Autodesk Inventor part; units mm, degrees
(part 2 of 3)
ref_plane "to_Bolt_1_28_YZ" through (-253.5817, 0, -380) normal (1, 0, 0) x (0, 0, -1)
ref_plane "to_Bolt_1_28_ZX" through (-253.5817, 0, -380) normal (0, 0, -1) x (0, 1, 0)
ref_plane "to_Bolt_1_29_XY" through (-251.8625, 0, -380) normal (0, 1, 0) x (1, 0, 0)
ref_plane "to_Bolt_1_29_YZ" through (-251.8625, 0, -380) normal (1, 0, 0) x (0, 0, -1)
ref_plane "to_Bolt_1_29_ZX" through (-251.8625, 0, -380) normal (0, 0, -1) x (0, 1, 0)
ref_plane "to_Bolt_1_3_XY" through (-296.5616, 0, -380) normal (0, 1, 0) x (1, 0, 0)
ref_plane "to_Bolt_1_3_YZ" through (-296.5616, 0, -380) normal (1, 0, 0) x (0, 0, -1)
ref_plane "to_Bolt_1_3_ZX" through (-296.5616, 0, -380) normal (0, 0, -1) x (0, 1, 0)
ref_plane "to_Bolt_1_30_XY" through (-250.1433, 0, -380) normal (0, 1, 0) x (1, 0, 0)
ref_plane "to_Bolt_1_30_YZ" through (-250.1433, 0, -380) normal (1, 0, 0) x (0, 0, -1)
ref_plane "to_Bolt_1_30_ZX" through (-250.1433, 0, -380) normal (0, 0, -1) x (0, 1, 0)
ref_plane "to_Bolt_1_31_XY" through (-248.4241, 0, -380) normal (0, 1, 0) x (1, 0, 0)
ref_plane "to_Bolt_1_31_YZ" through (-248.4241, 0, -380) normal (1, 0, 0) x (0, 0, -1)
ref_plane "to_Bolt_1_31_ZX" through (-248.4241, 0, -380) normal (0, 0, -1) x (0, 1, 0)
ref_plane "to_Bolt_1_32_XY" through (-246.7049, 0, -380) normal (0, 1, 0) x (1, 0, 0)
ref_plane "to_Bolt_1_32_YZ" through (-246.7049, 0, -380) normal (1, 0, 0) x (0, 0, -1)
ref_plane "to_Bolt_1_32_ZX" through (-246.7049, 0, -380) normal (0, 0, -1) x (0, 1, 0)
ref_plane "to_Bolt_1_33_XY" through (-244.9857, 0, -380) normal (0, 1, 0) x (1, 0, 0)
ref_plane "to_Bolt_1_33_YZ" through (-244.9857, 0, -380) normal (1, 0, 0) x (0, 0, -1)
ref_plane "to_Bolt_1_33_ZX" through (-244.9857, 0, -380) normal (0, 0, -1) x (0, 1, 0)
ref_plane "to_Bolt_1_34_XY" through (-243.2665, 0, -380) normal (0, 1, 0) x (1, 0, 0)
ref_plane "to_Bolt_1_34_YZ" through (-243.2665, 0, -380) normal (1, 0, 0) x (0, 0, -1)
ref_plane "to_Bolt_1_34_ZX" through (-243.2665, 0, -380) normal (0, 0, -1) x (0, 1, 0)
ref_plane "to_Bolt_1_35_XY" through (-241.5473, 0, -380) normal (0, 1, 0) x (1, 0, 0)
ref_plane "to_Bolt_1_35_YZ" through (-241.5473, 0, -380) normal (1, 0, 0) x (0, 0, -1)
ref_plane "to_Bolt_1_35_ZX" through (-241.5473, 0, -380) normal (0, 0, -1) x (0, 1, 0)
ref_plane "to_Bolt_1_352_XY" through (-134.957, 0, 380) normal (0, 1, 0) x (1, 0, 0)
ref_plane "to_Bolt_1_352_YZ" through (-134.957, 0, 380) normal (1, 0, 0) x (0, 0, -1)
ref_plane "to_Bolt_1_352_ZX" through (-134.957, 0, 380) normal (0, 0, -1) x (0, 1, 0)
ref_plane "to_Bolt_1_353_XY" through (-133.2378, 0, 380) normal (0, 1, 0) x (1, 0, 0)
ref_plane "to_Bolt_1_353_YZ" through (-133.2378, 0, 380) normal (1, 0, 0) x (0, 0, -1)
ref_plane "to_Bolt_1_353_ZX" through (-133.2378, 0, 380) normal (0, 0, -1) x (0, 1, 0)
ref_plane "to_Bolt_1_354_XY" through (-131.5186, 0, 380) normal (0, 1, 0) x (1, 0, 0)
ref_plane "to_Bolt_1_354_YZ" through (-131.5186, 0, 380) normal (1, 0, 0) x (0, 0, -1)
ref_plane "to_Bolt_1_354_ZX" through (-131.5186, 0, 380) normal (0, 0, -1) x (0, 1, 0)
ref_plane "to_Bolt_1_355_XY" through (-129.7994, 0, 380) normal (0, 1, 0) x (1, 0, 0)
ref_plane "to_Bolt_1_355_YZ" through (-129.7994, 0, 380) normal (1, 0, 0) x (0, 0, -1)
ref_plane "to_Bolt_1_355_ZX" through (-129.7994, 0, 380) normal (0, 0, -1) x (0, 1, 0)
ref_plane "to_Bolt_1_356_XY" through (-128.0802, 0, 380) normal (0, 1, 0) x (1, 0, 0)
ref_plane "to_Bolt_1_356_YZ" through (-128.0802, 0, 380) normal (1, 0, 0) x (0, 0, -1)
ref_plane "to_Bolt_1_356_ZX" through (-128.0802, 0, 380) normal (0, 0, -1) x (0, 1, 0)
ref_plane "to_Bolt_1_357_XY" through (-126.361, 0, 380) normal (0, 1, 0) x (1, 0, 0)
ref_plane "to_Bolt_1_357_YZ" through (-126.361, 0, 380) normal (1, 0, 0) x (0, 0, -1)
ref_plane "to_Bolt_1_357_ZX" through (-126.361, 0, 380) normal (0, 0, -1) x (0, 1, 0)
ref_plane "to_Bolt_1_358_XY" through (-124.6418, 0, 380) normal (0, 1, 0) x (1, 0, 0)
ref_plane "to_Bolt_1_358_YZ" through (-124.6418, 0, 380) normal (1, 0, 0) x (0, 0, -1)
ref_plane "to_Bolt_1_358_ZX" through (-124.6418, 0, 380) normal (0, 0, -1) x (0, 1, 0)
ref_plane "to_Bolt_1_359_XY" through (-122.9226, 0, 380) normal (0, 1, 0) x (1, 0, 0)
ref_plane "to_Bolt_1_359_YZ" through (-122.9226, 0, 380) normal (1, 0, 0) x (0, 0, -1)
ref_plane "to_Bolt_1_359_ZX" through (-122.9226, 0, 380) normal (0, 0, -1) x (0, 1, 0)
ref_plane "to_Bolt_1_36_XY" through (-239.8281, 0, -380) normal (0, 1, 0) x (1, 0, 0)
ref_plane "to_Bolt_1_36_YZ" through (-239.8281, 0, -380) normal (1, 0, 0) x (0, 0, -1)
ref_plane "to_Bolt_1_36_ZX" through (-239.8281, 0, -380) normal (0, 0, -1) x (0, 1, 0)
ref_plane "to_Bolt_1_360_XY" through (-121.2034, 0, 380) normal (0, 1, 0) x (1, 0, 0)
ref_plane "to_Bolt_1_360_YZ" through (-121.2034, 0, 380) normal (1, 0, 0) x (0, 0, -1)
ref_plane "to_Bolt_1_360_ZX" through (-121.2034, 0, 380) normal (0, 0, -1) x (0, 1, 0)
ref_plane "to_Bolt_1_361_XY" through (-119.4842, 0, 380) normal (0, 1, 0) x (1, 0, 0)
ref_plane "to_Bolt_1_361_YZ" through (-119.4842, 0, 380) normal (1, 0, 0) x (0, 0, -1)
ref_plane "to_Bolt_1_361_ZX" through (-119.4842, 0, 380) normal (0, 0, -1) x (0, 1, 0)
ref_plane "to_Bolt_1_362_XY" through (-117.765, 0, 380) normal (0, 1, 0) x (1, 0, 0)
ref_plane "to_Bolt_1_362_YZ" through (-117.765, 0, 380) normal (1, 0, 0) x (0, 0, -1)
ref_plane "to_Bolt_1_362_ZX" through (-117.765, 0, 380) normal (0, 0, -1) x (0, 1, 0)
ref_plane "to_Bolt_1_363_XY" through (-116.0458, 0, 380) normal (0, 1, 0) x (1, 0, 0)
ref_plane "to_Bolt_1_363_YZ" through (-116.0458, 0, 380) normal (1, 0, 0) x (0, 0, -1)
ref_plane "to_Bolt_1_363_ZX" through (-116.0458, 0, 380) normal (0, 0, -1) x (0, 1, 0)
ref_plane "to_Bolt_1_364_XY" through (-114.3266, 0, 380) normal (0, 1, 0) x (1, 0, 0)
ref_plane "to_Bolt_1_364_YZ" through (-114.3266, 0, 380) normal (1, 0, 0) x (0, 0, -1)
ref_plane "to_Bolt_1_364_ZX" through (-114.3266, 0, 380) normal (0, 0, -1) x (0, 1, 0)
ref_plane "to_Bolt_1_365_XY" through (-112.6074, 0, 380) normal (0, 1, 0) x (1, 0, 0)
ref_plane "to_Bolt_1_365_YZ" through (-112.6074, 0, 380) normal (1, 0, 0) x (0, 0, -1)
ref_plane "to_Bolt_1_365_ZX" through (-112.6074, 0, 380) normal (0, 0, -1) x (0, 1, 0)
ref_plane "to_Bolt_1_366_XY" through (-110.8883, 0, 380) normal (0, 1, 0) x (1, 0, 0)
ref_plane "to_Bolt_1_366_YZ" through (-110.8883, 0, 380) normal (1, 0, 0) x (0, 0, -1)
ref_plane "to_Bolt_1_366_ZX" through (-110.8883, 0, 380) normal (0, 0, -1) x (0, 1, 0)
ref_plane "to_Bolt_1_367_XY" through (-109.1691, 0, 380) normal (0, 1, 0) x (1, 0, 0)
ref_plane "to_Bolt_1_367_YZ" through (-109.1691, 0, 380) normal (1, 0, 0) x (0, 0, -1)
ref_plane "to_Bolt_1_367_ZX" through (-109.1691, 0, 380) normal (0, 0, -1) x (0, 1, 0)
ref_plane "to_Bolt_1_368_XY" through (-107.4499, 0, 380) normal (0, 1, 0) x (1, 0, 0)
ref_plane "to_Bolt_1_368_YZ" through (-107.4499, 0, 380) normal (1, 0, 0) x (0, 0, -1)
ref_plane "to_Bolt_1_368_ZX" through (-107.4499, 0, 380) normal (0, 0, -1) x (0, 1, 0)
ref_plane "to_Bolt_1_369_XY" through (-105.7307, 0, 380) normal (0, 1, 0) x (1, 0, 0)
ref_plane "to_Bolt_1_369_YZ" through (-105.7307, 0, 380) normal (1, 0, 0) x (0, 0, -1)
ref_plane "to_Bolt_1_369_ZX" through (-105.7307, 0, 380) normal (0, 0, -1) x (0, 1, 0)
ref_plane "to_Bolt_1_37_XY" through (-238.1089, 0, -380) normal (0, 1, 0) x (1, 0, 0)
ref_plane "to_Bolt_1_37_YZ" through (-238.1089, 0, -380) normal (1, 0, 0) x (0, 0, -1)
ref_plane "to_Bolt_1_37_ZX" through (-238.1089, 0, -380) normal (0, 0, -1) x (0, 1, 0)
ref_plane "to_Bolt_1_370_XY" through (-104.0115, 0, 380) normal (0, 1, 0) x (1, 0, 0)
ref_plane "to_Bolt_1_370_YZ" through (-104.0115, 0, 380) normal (1, 0, 0) x (0, 0, -1)
ref_plane "to_Bolt_1_370_ZX" through (-104.0115, 0, 380) normal (0, 0, -1) x (0, 1, 0)
ref_plane "to_Bolt_1_371_XY" through (-102.2923, 0, 380) normal (0, 1, 0) x (1, 0, 0)
ref_plane "to_Bolt_1_371_YZ" through (-102.2923, 0, 380) normal (1, 0, 0) x (0, 0, -1)
ref_plane "to_Bolt_1_371_ZX" through (-102.2923, 0, 380) normal (0, 0, -1) x (0, 1, 0)
ref_plane "to_Bolt_1_372_XY" through (-100.5731, 0, 380) normal (0, 1, 0) x (1, 0, 0)
ref_plane "to_Bolt_1_372_YZ" through (-100.5731, 0, 380) normal (1, 0, 0) x (0, 0, -1)
ref_plane "to_Bolt_1_372_ZX" through (-100.5731, 0, 380) normal (0, 0, -1) x (0, 1, 0)
ref_plane "to_Bolt_1_373_XY" through (-98.8539, 0, 380) normal (0, 1, 0) x (1, 0, 0)
ref_plane "to_Bolt_1_373_YZ" through (-98.8539, 0, 380) normal (1, 0, 0) x (0, 0, -1)
ref_plane "to_Bolt_1_373_ZX" through (-98.8539, 0, 380) normal (0, 0, -1) x (0, 1, 0)
ref_plane "to_Bolt_1_374_XY" through (-97.1347, 0, 380) normal (0, 1, 0) x (1, 0, 0)
ref_plane "to_Bolt_1_374_YZ" through (-97.1347, 0, 380) normal (1, 0, 0) x (0, 0, -1)
ref_plane "to_Bolt_1_374_ZX" through (-97.1347, 0, 380) normal (0, 0, -1) x (0, 1, 0)
ref_plane "to_Bolt_1_375_XY" through (-95.4155, 0, 380) normal (0, 1, 0) x (1, 0, 0)
ref_plane "to_Bolt_1_375_YZ" through (-95.4155, 0, 380) normal (1, 0, 0) x (0, 0, -1)
ref_plane "to_Bolt_1_375_ZX" through (-95.4155, 0, 380) normal (0, 0, -1) x (0, 1, 0)
ref_plane "to_Bolt_1_376_XY" through (-93.6963, 0, 380) normal (0, 1, 0) x (1, 0, 0)
ref_plane "to_Bolt_1_376_YZ" through (-93.6963, 0, 380) normal (1, 0, 0) x (0, 0, -1)
ref_plane "to_Bolt_1_376_ZX" through (-93.6963, 0, 380) normal (0, 0, -1) x (0, 1, 0)
ref_plane "to_Bolt_1_377_XY" through (-91.9771, 0, 380) normal (0, 1, 0) x (1, 0, 0)
ref_plane "to_Bolt_1_377_YZ" through (-91.9771, 0, 380) normal (1, 0, 0) x (0, 0, -1)
ref_plane "to_Bolt_1_377_ZX" through (-91.9771, 0, 380) normal (0, 0, -1) x (0, 1, 0)
ref_plane "to_Bolt_1_378_XY" through (-90.2579, 0, 380) normal (0, 1, 0) x (1, 0, 0)
ref_plane "to_Bolt_1_378_YZ" through (-90.2579, 0, 380) normal (1, 0, 0) x (0, 0, -1)
ref_plane "to_Bolt_1_378_ZX" through (-90.2579, 0, 380) normal (0, 0, -1) x (0, 1, 0)
ref_plane "to_Bolt_1_379_XY" through (-88.5387, 0, 380) normal (0, 1, 0) x (1, 0, 0)
ref_plane "to_Bolt_1_379_YZ" through (-88.5387, 0, 380) normal (1, 0, 0) x (0, 0, -1)
ref_plane "to_Bolt_1_379_ZX" through (-88.5387, 0, 380) normal (0, 0, -1) x (0, 1, 0)
ref_plane "to_Bolt_1_38_XY" through (-236.3897, 0, -380) normal (0, 1, 0) x (1, 0, 0)
ref_plane "to_Bolt_1_38_YZ" through (-236.3897, 0, -380) normal (1, 0, 0) x (0, 0, -1)
ref_plane "to_Bolt_1_38_ZX" through (-236.3897, 0, -380) normal (0, 0, -1) x (0, 1, 0)
ref_plane "to_Bolt_1_380_XY" through (-86.8195, 0, 380) normal (0, 1, 0) x (1, 0, 0)
ref_plane "to_Bolt_1_380_YZ" through (-86.8195, 0, 380) normal (1, 0, 0) x (0, 0, -1)
ref_plane "to_Bolt_1_380_ZX" through (-86.8195, 0, 380) normal (0, 0, -1) x (0, 1, 0)
ref_plane "to_Bolt_1_381_XY" through (-85.1003, 0, 380) normal (0, 1, 0) x (1, 0, 0)
ref_plane "to_Bolt_1_381_YZ" through (-85.1003, 0, 380) normal (1, 0, 0) x (0, 0, -1)
ref_plane "to_Bolt_1_381_ZX" through (-85.1003, 0, 380) normal (0, 0, -1) x (0, 1, 0)
ref_plane "to_Bolt_1_382_XY" through (-83.3811, 0, 380) normal (0, 1, 0) x (1, 0, 0)
ref_plane "to_Bolt_1_382_YZ" through (-83.3811, 0, 380) normal (1, 0, 0) x (0, 0, -1)
ref_plane "to_Bolt_1_382_ZX" through (-83.3811, 0, 380) normal (0, 0, -1) x (0, 1, 0)
ref_plane "to_Bolt_1_383_XY" through (-81.6619, 0, 380) normal (0, 1, 0) x (1, 0, 0)
ref_plane "to_Bolt_1_383_YZ" through (-81.6619, 0, 380) normal (1, 0, 0) x (0, 0, -1)
ref_plane "to_Bolt_1_383_ZX" through (-81.6619, 0, 380) normal (0, 0, -1) x (0, 1, 0)
ref_plane "to_Bolt_1_384_XY" through (-79.9427, 0, 380) normal (0, 1, 0) x (1, 0, 0)
ref_plane "to_Bolt_1_384_YZ" through (-79.9427, 0, 380) normal (1, 0, 0) x (0, 0, -1)
ref_plane "to_Bolt_1_384_ZX" through (-79.9427, 0, 380) normal (0, 0, -1) x (0, 1, 0)
ref_plane "to_Bolt_1_385_XY" through (-78.2235, 0, 380) normal (0, 1, 0) x (1, 0, 0)
ref_plane "to_Bolt_1_385_YZ" through (-78.2235, 0, 380) normal (1, 0, 0) x (0, 0, -1)
ref_plane "to_Bolt_1_385_ZX" through (-78.2235, 0, 380) normal (0, 0, -1) x (0, 1, 0)
ref_plane "to_Bolt_1_386_XY" through (-76.5043, 0, 380) normal (0, 1, 0) x (1, 0, 0)
ref_plane "to_Bolt_1_386_YZ" through (-76.5043, 0, 380) normal (1, 0, 0) x (0, 0, -1)
ref_plane "to_Bolt_1_386_ZX" through (-76.5043, 0, 380) normal (0, 0, -1) x (0, 1, 0)
ref_plane "to_Bolt_1_387_XY" through (-74.7851, 0, 380) normal (0, 1, 0) x (1, 0, 0)
ref_plane "to_Bolt_1_387_YZ" through (-74.7851, 0, 380) normal (1, 0, 0) x (0, 0, -1)
ref_plane "to_Bolt_1_387_ZX" through (-74.7851, 0, 380) normal (0, 0, -1) x (0, 1, 0)
ref_plane "to_Bolt_1_388_XY" through (-73.0659, 0, 380) normal (0, 1, 0) x (1, 0, 0)
ref_plane "to_Bolt_1_388_YZ" through (-73.0659, 0, 380) normal (1, 0, 0) x (0, 0, -1)
ref_plane "to_Bolt_1_388_ZX" through (-73.0659, 0, 380) normal (0, 0, -1) x (0, 1, 0)
ref_plane "to_Bolt_1_389_XY" through (-71.3467, 0, 380) normal (0, 1, 0) x (1, 0, 0)
ref_plane "to_Bolt_1_389_YZ" through (-71.3467, 0, 380) normal (1, 0, 0) x (0, 0, -1)
ref_plane "to_Bolt_1_389_ZX" through (-71.3467, 0, 380) normal (0, 0, -1) x (0, 1, 0)
ref_plane "to_Bolt_1_39_XY" through (-234.6705, 0, -380) normal (0, 1, 0) x (1, 0, 0)
ref_plane "to_Bolt_1_39_YZ" through (-234.6705, 0, -380) normal (1, 0, 0) x (0, 0, -1)
ref_plane "to_Bolt_1_39_ZX" through (-234.6705, 0, -380) normal (0, 0, -1) x (0, 1, 0)
ref_plane "to_Bolt_1_390_XY" through (-69.6275, 0, 380) normal (0, 1, 0) x (1, 0, 0)
ref_plane "to_Bolt_1_390_YZ" through (-69.6275, 0, 380) normal (1, 0, 0) x (0, 0, -1)
ref_plane "to_Bolt_1_390_ZX" through (-69.6275, 0, 380) normal (0, 0, -1) x (0, 1, 0)
ref_plane "to_Bolt_1_391_XY" through (-67.9083, 0, 380) normal (0, 1, 0) x (1, 0, 0)
ref_plane "to_Bolt_1_391_YZ" through (-67.9083, 0, 380) normal (1, 0, 0) x (0, 0, -1)
ref_plane "to_Bolt_1_391_ZX" through (-67.9083, 0, 380) normal (0, 0, -1) x (0, 1, 0)
ref_plane "to_Bolt_1_392_XY" through (-66.1891, 0, 380) normal (0, 1, 0) x (1, 0, 0)
ref_plane "to_Bolt_1_392_YZ" through (-66.1891, 0, 380) normal (1, 0, 0) x (0, 0, -1)
ref_plane "to_Bolt_1_392_ZX" through (-66.1891, 0, 380) normal (0, 0, -1) x (0, 1, 0)
ref_plane "to_Bolt_1_393_XY" through (-64.4699, 0, 380) normal (0, 1, 0) x (1, 0, 0)
ref_plane "to_Bolt_1_393_YZ" through (-64.4699, 0, 380) normal (1, 0, 0) x (0, 0, -1)
ref_plane "to_Bolt_1_393_ZX" through (-64.4699, 0, 380) normal (0, 0, -1) x (0, 1, 0)
ref_plane "to_Bolt_1_394_XY" through (-62.7507, 0, 380) normal (0, 1, 0) x (1, 0, 0)
ref_plane "to_Bolt_1_394_YZ" through (-62.7507, 0, 380) normal (1, 0, 0) x (0, 0, -1)
ref_plane "to_Bolt_1_394_ZX" through (-62.7507, 0, 380) normal (0, 0, -1) x (0, 1, 0)
ref_plane "to_Bolt_1_395_XY" through (-61.0315, 0, 380) normal (0, 1, 0) x (1, 0, 0)
ref_plane "to_Bolt_1_395_YZ" through (-61.0315, 0, 380) normal (1, 0, 0) x (0, 0, -1)
ref_plane "to_Bolt_1_395_ZX" through (-61.0315, 0, 380) normal (0, 0, -1) x (0, 1, 0)
ref_plane "to_Bolt_1_396_XY" through (-59.3123, 0, 380) normal (0, 1, 0) x (1, 0, 0)
ref_plane "to_Bolt_1_396_YZ" through (-59.3123, 0, 380) normal (1, 0, 0) x (0, 0, -1)
ref_plane "to_Bolt_1_396_ZX" through (-59.3123, 0, 380) normal (0, 0, -1) x (0, 1, 0)
ref_plane "to_Bolt_1_397_XY" through (-57.5931, 0, 380) normal (0, 1, 0) x (1, 0, 0)
ref_plane "to_Bolt_1_397_YZ" through (-57.5931, 0, 380) normal (1, 0, 0) x (0, 0, -1)
ref_plane "to_Bolt_1_397_ZX" through (-57.5931, 0, 380) normal (0, 0, -1) x (0, 1, 0)
ref_plane "to_Bolt_1_398_XY" through (-55.8739, 0, 380) normal (0, 1, 0) x (1, 0, 0)
ref_plane "to_Bolt_1_398_YZ" through (-55.8739, 0, 380) normal (1, 0, 0) x (0, 0, -1)
ref_plane "to_Bolt_1_398_ZX" through (-55.8739, 0, 380) normal (0, 0, -1) x (0, 1, 0)
ref_plane "to_Bolt_1_399_XY" through (-54.1547, 0, 380) normal (0, 1, 0) x (1, 0, 0)
ref_plane "to_Bolt_1_399_YZ" through (-54.1547, 0, 380) normal (1, 0, 0) x (0, 0, -1)
ref_plane "to_Bolt_1_399_ZX" through (-54.1547, 0, 380) normal (0, 0, -1) x (0, 1, 0)
ref_plane "to_Bolt_1_4_XY" through (-294.8424, 0, -380) normal (0, 1, 0) x (1, 0, 0)
ref_plane "to_Bolt_1_4_YZ" through (-294.8424, 0, -380) normal (1, 0, 0) x (0, 0, -1)
ref_plane "to_Bolt_1_4_ZX" through (-294.8424, 0, -380) normal (0, 0, -1) x (0, 1, 0)
ref_plane "to_Bolt_1_40_XY" through (-232.9513, 0, -380) normal (0, 1, 0) x (1, 0, 0)
ref_plane "to_Bolt_1_40_YZ" through (-232.9513, 0, -380) normal (1, 0, 0) x (0, 0, -1)
ref_plane "to_Bolt_1_40_ZX" through (-232.9513, 0, -380) normal (0, 0, -1) x (0, 1, 0)
ref_plane "to_Bolt_1_400_XY" through (-52.4355, 0, 380) normal (0, 1, 0) x (1, 0, 0)
ref_plane "to_Bolt_1_400_YZ" through (-52.4355, 0, 380) normal (1, 0, 0) x (0, 0, -1)
ref_plane "to_Bolt_1_400_ZX" through (-52.4355, 0, 380) normal (0, 0, -1) x (0, 1, 0)
ref_plane "to_Bolt_1_401_XY" through (-50.7163, 0, 380) normal (0, 1, 0) x (1, 0, 0)
ref_plane "to_Bolt_1_401_YZ" through (-50.7163, 0, 380) normal (1, 0, 0) x (0, 0, -1)
ref_plane "to_Bolt_1_401_ZX" through (-50.7163, 0, 380) normal (0, 0, -1) x (0, 1, 0)
ref_plane "to_Bolt_1_402_XY" through (-48.9971, 0, 380) normal (0, 1, 0) x (1, 0, 0)
ref_plane "to_Bolt_1_402_YZ" through (-48.9971, 0, 380) normal (1, 0, 0) x (0, 0, -1)
ref_plane "to_Bolt_1_402_ZX" through (-48.9971, 0, 380) normal (0, 0, -1) x (0, 1, 0)
ref_plane "to_Bolt_1_403_XY" through (-47.2779, 0, 380) normal (0, 1, 0) x (1, 0, 0)
ref_plane "to_Bolt_1_403_YZ" through (-47.2779, 0, 380) normal (1, 0, 0) x (0, 0, -1)
ref_plane "to_Bolt_1_403_ZX" through (-47.2779, 0, 380) normal (0, 0, -1) x (0, 1, 0)
ref_plane "to_Bolt_1_404_XY" through (-45.5587, 0, 380) normal (0, 1, 0) x (1, 0, 0)
ref_plane "to_Bolt_1_404_YZ" through (-45.5587, 0, 380) normal (1, 0, 0) x (0, 0, -1)
ref_plane "to_Bolt_1_404_ZX" through (-45.5587, 0, 380) normal (0, 0, -1) x (0, 1, 0)
ref_plane "to_Bolt_1_405_XY" through (-43.8395, 0, 380) normal (0, 1, 0) x (1, 0, 0)
ref_plane "to_Bolt_1_405_YZ" through (-43.8395, 0, 380) normal (1, 0, 0) x (0, 0, -1)
ref_plane "to_Bolt_1_405_ZX" through (-43.8395, 0, 380) normal (0, 0, -1) x (0, 1, 0)
ref_plane "to_Bolt_1_406_XY" through (-42.1203, 0, 380) normal (0, 1, 0) x (1, 0, 0)
ref_plane "to_Bolt_1_406_YZ" through (-42.1203, 0, 380) normal (1, 0, 0) x (0, 0, -1)
ref_plane "to_Bolt_1_406_ZX" through (-42.1203, 0, 380) normal (0, 0, -1) x (0, 1, 0)
ref_plane "to_Bolt_1_407_XY" through (-40.4011, 0, 380) normal (0, 1, 0) x (1, 0, 0)
ref_plane "to_Bolt_1_407_YZ" through (-40.4011, 0, 380) normal (1, 0, 0) x (0, 0, -1)
ref_plane "to_Bolt_1_407_ZX" through (-40.4011, 0, 380) normal (0, 0, -1) x (0, 1, 0)
ref_plane "to_Bolt_1_408_XY" through (-38.6819, 0, 380) normal (0, 1, 0) x (1, 0, 0)
ref_plane "to_Bolt_1_408_YZ" through (-38.6819, 0, 380) normal (1, 0, 0) x (0, 0, -1)
ref_plane "to_Bolt_1_408_ZX" through (-38.6819, 0, 380) normal (0, 0, -1) x (0, 1, 0)
ref_plane "to_Bolt_1_409_XY" through (-36.9628, 0, 380) normal (0, 1, 0) x (1, 0, 0)
ref_plane "to_Bolt_1_409_YZ" through (-36.9628, 0, 380) normal (1, 0, 0) x (0, 0, -1)
ref_plane "to_Bolt_1_409_ZX" through (-36.9628, 0, 380) normal (0, 0, -1) x (0, 1, 0)
ref_plane "to_Bolt_1_41_XY" through (-231.2321, 0, -380) normal (0, 1, 0) x (1, 0, 0)
ref_plane "to_Bolt_1_41_YZ" through (-231.2321, 0, -380) normal (1, 0, 0) x (0, 0, -1)
ref_plane "to_Bolt_1_41_ZX" through (-231.2321, 0, -380) normal (0, 0, -1) x (0, 1, 0)
ref_plane "to_Bolt_1_410_XY" through (-35.2436, 0, 380) normal (0, 1, 0) x (1, 0, 0)
ref_plane "to_Bolt_1_410_YZ" through (-35.2436, 0, 380) normal (1, 0, 0) x (0, 0, -1)
ref_plane "to_Bolt_1_410_ZX" through (-35.2436, 0, 380) normal (0, 0, -1) x (0, 1, 0)
ref_plane "to_Bolt_1_411_XY" through (-33.5244, 0, 380) normal (0, 1, 0) x (1, 0, 0)
ref_plane "to_Bolt_1_411_YZ" through (-33.5244, 0, 380) normal (1, 0, 0) x (0, 0, -1)
ref_plane "to_Bolt_1_411_ZX" through (-33.5244, 0, 380) normal (0, 0, -1) x (0, 1, 0)
ref_plane "to_Bolt_1_412_XY" through (-31.8052, 0, 380) normal (0, 1, 0) x (1, 0, 0)
ref_plane "to_Bolt_1_412_YZ" through (-31.8052, 0, 380) normal (1, 0, 0) x (0, 0, -1)
ref_plane "to_Bolt_1_412_ZX" through (-31.8052, 0, 380) normal (0, 0, -1) x (0, 1, 0)
ref_plane "to_Bolt_1_413_XY" through (-30.086, 0, 380) normal (0, 1, 0) x (1, 0, 0)
ref_plane "to_Bolt_1_413_YZ" through (-30.086, 0, 380) normal (1, 0, 0) x (0, 0, -1)
ref_plane "to_Bolt_1_413_ZX" through (-30.086, 0, 380) normal (0, 0, -1) x (0, 1, 0)
ref_plane "to_Bolt_1_414_XY" through (-28.3668, 0, 380) normal (0, 1, 0) x (1, 0, 0)
ref_plane "to_Bolt_1_414_YZ" through (-28.3668, 0, 380) normal (1, 0, 0) x (0, 0, -1)
ref_plane "to_Bolt_1_414_ZX" through (-28.3668, 0, 380) normal (0, 0, -1) x (0, 1, 0)
ref_plane "to_Bolt_1_415_XY" through (-26.6476, 0, 380) normal (0, 1, 0) x (1, 0, 0)
ref_plane "to_Bolt_1_415_YZ" through (-26.6476, 0, 380) normal (1, 0, 0) x (0, 0, -1)
ref_plane "to_Bolt_1_415_ZX" through (-26.6476, 0, 380) normal (0, 0, -1) x (0, 1, 0)
ref_plane "to_Bolt_1_416_XY" through (-24.9284, 0, 380) normal (0, 1, 0) x (1, 0, 0)
ref_plane "to_Bolt_1_416_YZ" through (-24.9284, 0, 380) normal (1, 0, 0) x (0, 0, -1)
ref_plane "to_Bolt_1_416_ZX" through (-24.9284, 0, 380) normal (0, 0, -1) x (0, 1, 0)
ref_plane "to_Bolt_1_417_XY" through (-23.2092, 0, 380) normal (0, 1, 0) x (1, 0, 0)
ref_plane "to_Bolt_1_417_YZ" through (-23.2092, 0, 380) normal (1, 0, 0) x (0, 0, -1)
ref_plane "to_Bolt_1_417_ZX" through (-23.2092, 0, 380) normal (0, 0, -1) x (0, 1, 0)
ref_plane "to_Bolt_1_418_XY" through (-21.49, 0, 380) normal (0, 1, 0) x (1, 0, 0)
ref_plane "to_Bolt_1_418_YZ" through (-21.49, 0, 380) normal (1, 0, 0) x (0, 0, -1)
ref_plane "to_Bolt_1_418_ZX" through (-21.49, 0, 380) normal (0, 0, -1) x (0, 1, 0)
ref_plane "to_Bolt_1_419_XY" through (-19.7708, 0, 380) normal (0, 1, 0) x (1, 0, 0)
ref_plane "to_Bolt_1_419_YZ" through (-19.7708, 0, 380) normal (1, 0, 0) x (0, 0, -1)
ref_plane "to_Bolt_1_419_ZX" through (-19.7708, 0, 380) normal (0, 0, -1) x (0, 1, 0)
ref_plane "to_Bolt_1_42_XY" through (-229.5129, 0, -380) normal (0, 1, 0) x (1, 0, 0)
ref_plane "to_Bolt_1_42_YZ" through (-229.5129, 0, -380) normal (1, 0, 0) x (0, 0, -1)
ref_plane "to_Bolt_1_42_ZX" through (-229.5129, 0, -380) normal (0, 0, -1) x (0, 1, 0)
ref_plane "to_Bolt_1_420_XY" through (-18.0516, 0, 380) normal (0, 1, 0) x (1, 0, 0)
ref_plane "to_Bolt_1_420_YZ" through (-18.0516, 0, 380) normal (1, 0, 0) x (0, 0, -1)
ref_plane "to_Bolt_1_420_ZX" through (-18.0516, 0, 380) normal (0, 0, -1) x (0, 1, 0)
ref_plane "to_Bolt_1_421_XY" through (-16.3324, 0, 380) normal (0, 1, 0) x (1, 0, 0)
ref_plane "to_Bolt_1_421_YZ" through (-16.3324, 0, 380) normal (1, 0, 0) x (0, 0, -1)
ref_plane "to_Bolt_1_421_ZX" through (-16.3324, 0, 380) normal (0, 0, -1) x (0, 1, 0)
ref_plane "to_Bolt_1_422_XY" through (-14.6132, 0, 380) normal (0, 1, 0) x (1, 0, 0)
ref_plane "to_Bolt_1_422_YZ" through (-14.6132, 0, 380) normal (1, 0, 0) x (0, 0, -1)
ref_plane "to_Bolt_1_422_ZX" through (-14.6132, 0, 380) normal (0, 0, -1) x (0, 1, 0)
ref_plane "to_Bolt_1_423_XY" through (-12.894, 0, 380) normal (0, 1, 0) x (1, 0, 0)
ref_plane "to_Bolt_1_423_YZ" through (-12.894, 0, 380) normal (1, 0, 0) x (0, 0, -1)
ref_plane "to_Bolt_1_423_ZX" through (-12.894, 0, 380) normal (0, 0, -1) x (0, 1, 0)
ref_plane "to_Bolt_1_424_XY" through (-11.1748, 0, 380) normal (0, 1, 0) x (1, 0, 0)
ref_plane "to_Bolt_1_424_YZ" through (-11.1748, 0, 380) normal (1, 0, 0) x (0, 0, -1)
ref_plane "to_Bolt_1_424_ZX" through (-11.1748, 0, 380) normal (0, 0, -1) x (0, 1, 0)
ref_plane "to_Bolt_1_425_XY" through (-9.4556, 0, 380) normal (0, 1, 0) x (1, 0, 0)
ref_plane "to_Bolt_1_425_YZ" through (-9.4556, 0, 380) normal (1, 0, 0) x (0, 0, -1)
ref_plane "to_Bolt_1_425_ZX" through (-9.4556, 0, 380) normal (0, 0, -1) x (0, 1, 0)
ref_plane "to_Bolt_1_426_XY" through (-7.7364, 0, 380) normal (0, 1, 0) x (1, 0, 0)
ref_plane "to_Bolt_1_426_YZ" through (-7.7364, 0, 380) normal (1, 0, 0) x (0, 0, -1)
ref_plane "to_Bolt_1_426_ZX" through (-7.7364, 0, 380) normal (0, 0, -1) x (0, 1, 0)
ref_plane "to_Bolt_1_427_XY" through (-6.0172, 0, 380) normal (0, 1, 0) x (1, 0, 0)
ref_plane "to_Bolt_1_427_YZ" through (-6.0172, 0, 380) normal (1, 0, 0) x (0, 0, -1)
ref_plane "to_Bolt_1_427_ZX" through (-6.0172, 0, 380) normal (0, 0, -1) x (0, 1, 0)
ref_plane "to_Bolt_1_428_XY" through (-4.298, 0, 380) normal (0, 1, 0) x (1, 0, 0)
ref_plane "to_Bolt_1_428_YZ" through (-4.298, 0, 380) normal (1, 0, 0) x (0, 0, -1)
ref_plane "to_Bolt_1_428_ZX" through (-4.298, 0, 380) normal (0, 0, -1) x (0, 1, 0)
ref_plane "to_Bolt_1_429_XY" through (-2.5788, 0, 380) normal (0, 1, 0) x (1, 0, 0)
ref_plane "to_Bolt_1_429_YZ" through (-2.5788, 0, 380) normal (1, 0, 0) x (0, 0, -1)
ref_plane "to_Bolt_1_429_ZX" through (-2.5788, 0, 380) normal (0, 0, -1) x (0, 1, 0)
ref_plane "to_Bolt_1_43_XY" through (-227.7937, 0, -380) normal (0, 1, 0) x (1, 0, 0)
ref_plane "to_Bolt_1_43_YZ" through (-227.7937, 0, -380) normal (1, 0, 0) x (0, 0, -1)
ref_plane "to_Bolt_1_43_ZX" through (-227.7937, 0, -380) normal (0, 0, -1) x (0, 1, 0)
ref_plane "to_Bolt_1_430_XY" through (-0.8596, 0, 380) normal (0, 1, 0) x (1, 0, 0)
ref_plane "to_Bolt_1_430_YZ" through (-0.8596, 0, 380) normal (1, 0, 0) x (0, 0, -1)
ref_plane "to_Bolt_1_430_ZX" through (-0.8596, 0, 380) normal (0, 0, -1) x (0, 1, 0)
ref_plane "to_Bolt_1_431_XY" through (0.8596, 0, 380) normal (0, 1, 0) x (1, 0, 0)
ref_plane "to_Bolt_1_431_YZ" through (0.8596, 0, 380) normal (1, 0, 0) x (0, 0, -1)
ref_plane "to_Bolt_1_431_ZX" through (0.8596, 0, 380) normal (0, 0, -1) x (0, 1, 0)
ref_plane "to_Bolt_1_432_XY" through (2.5788, 0, 380) normal (0, 1, 0) x (1, 0, 0)
ref_plane "to_Bolt_1_432_YZ" through (2.5788, 0, 380) normal (1, 0, 0) x (0, 0, -1)
ref_plane "to_Bolt_1_432_ZX" through (2.5788, 0, 380) normal (0, 0, -1) x (0, 1, 0)
ref_plane "to_Bolt_1_433_XY" through (4.298, 0, 380) normal (0, 1, 0) x (1, 0, 0)
ref_plane "to_Bolt_1_433_YZ" through (4.298, 0, 380) normal (1, 0, 0) x (0, 0, -1)
ref_plane "to_Bolt_1_433_ZX" through (4.298, 0, 380) normal (0, 0, -1) x (0, 1, 0)
ref_plane "to_Bolt_1_434_XY" through (6.0172, 0, 380) normal (0, 1, 0) x (1, 0, 0)
ref_plane "to_Bolt_1_434_YZ" through (6.0172, 0, 380) normal (1, 0, 0) x (0, 0, -1)
ref_plane "to_Bolt_1_434_ZX" through (6.0172, 0, 380) normal (0, 0, -1) x (0, 1, 0)
ref_plane "to_Bolt_1_435_XY" through (7.7364, 0, 380) normal (0, 1, 0) x (1, 0, 0)
ref_plane "to_Bolt_1_435_YZ" through (7.7364, 0, 380) normal (1, 0, 0) x (0, 0, -1)
ref_plane "to_Bolt_1_435_ZX" through (7.7364, 0, 380) normal (0, 0, -1) x (0, 1, 0)
ref_plane "to_Bolt_1_436_XY" through (9.4556, 0, 380) normal (0, 1, 0) x (1, 0, 0)
ref_plane "to_Bolt_1_436_YZ" through (9.4556, 0, 380) normal (1, 0, 0) x (0, 0, -1)
ref_plane "to_Bolt_1_436_ZX" through (9.4556, 0, 380) normal (0, 0, -1) x (0, 1, 0)
ref_plane "to_Bolt_1_437_XY" through (11.1748, 0, 380) normal (0, 1, 0) x (1, 0, 0)
ref_plane "to_Bolt_1_437_YZ" through (11.1748, 0, 380) normal (1, 0, 0) x (0, 0, -1)
ref_plane "to_Bolt_1_437_ZX" through (11.1748, 0, 380) normal (0, 0, -1) x (0, 1, 0)
ref_plane "to_Bolt_1_438_XY" through (12.894, 0, 380) normal (0, 1, 0) x (1, 0, 0)
ref_plane "to_Bolt_1_438_YZ" through (12.894, 0, 380) normal (1, 0, 0) x (0, 0, -1)
ref_plane "to_Bolt_1_438_ZX" through (12.894, 0, 380) normal (0, 0, -1) x (0, 1, 0)
ref_plane "to_Bolt_1_439_XY" through (14.6132, 0, 380) normal (0, 1, 0) x (1, 0, 0)
ref_plane "to_Bolt_1_439_YZ" through (14.6132, 0, 380) normal (1, 0, 0) x (0, 0, -1)
ref_plane "to_Bolt_1_439_ZX" through (14.6132, 0, 380) normal (0, 0, -1) x (0, 1, 0)
ref_plane "to_Bolt_1_44_XY" through (-226.0745, 0, -380) normal (0, 1, 0) x (1, 0, 0)
ref_plane "to_Bolt_1_44_YZ" through (-226.0745, 0, -380) normal (1, 0, 0) x (0, 0, -1)
ref_plane "to_Bolt_1_44_ZX" through (-226.0745, 0, -380) normal (0, 0, -1) x (0, 1, 0)
ref_plane "to_Bolt_1_440_XY" through (16.3324, 0, 380) normal (0, 1, 0) x (1, 0, 0)
ref_plane "to_Bolt_1_440_YZ" through (16.3324, 0, 380) normal (1, 0, 0) x (0, 0, -1)
ref_plane "to_Bolt_1_440_ZX" through (16.3324, 0, 380) normal (0, 0, -1) x (0, 1, 0)
ref_plane "to_Bolt_1_441_XY" through (18.0516, 0, 380) normal (0, 1, 0) x (1, 0, 0)
ref_plane "to_Bolt_1_441_YZ" through (18.0516, 0, 380) normal (1, 0, 0) x (0, 0, -1)
ref_plane "to_Bolt_1_441_ZX" through (18.0516, 0, 380) normal (0, 0, -1) x (0, 1, 0)
ref_plane "to_Bolt_1_442_XY" through (19.7708, 0, 380) normal (0, 1, 0) x (1, 0, 0)
ref_plane "to_Bolt_1_442_YZ" through (19.7708, 0, 380) normal (1, 0, 0) x (0, 0, -1)
ref_plane "to_Bolt_1_442_ZX" through (19.7708, 0, 380) normal (0, 0, -1) x (0, 1, 0)
ref_plane "to_Bolt_1_443_XY" through (21.49, 0, 380) normal (0, 1, 0) x (1, 0, 0)
ref_plane "to_Bolt_1_443_YZ" through (21.49, 0, 380) normal (1, 0, 0) x (0, 0, -1)
ref_plane "to_Bolt_1_443_ZX" through (21.49, 0, 380) normal (0, 0, -1) x (0, 1, 0)
ref_plane "to_Bolt_1_444_XY" through (23.2092, 0, 380) normal (0, 1, 0) x (1, 0, 0)
ref_plane "to_Bolt_1_444_YZ" through (23.2092, 0, 380) normal (1, 0, 0) x (0, 0, -1)
ref_plane "to_Bolt_1_444_ZX" through (23.2092, 0, 380) normal (0, 0, -1) x (0, 1, 0)
ref_plane "to_Bolt_1_445_XY" through (24.9284, 0, 380) normal (0, 1, 0) x (1, 0, 0)
ref_plane "to_Bolt_1_445_YZ" through (24.9284, 0, 380) normal (1, 0, 0) x (0, 0, -1)
ref_plane "to_Bolt_1_445_ZX" through (24.9284, 0, 380) normal (0, 0, -1) x (0, 1, 0)
ref_plane "to_Bolt_1_446_XY" through (26.6476, 0, 380) normal (0, 1, 0) x (1, 0, 0)
ref_plane "to_Bolt_1_446_YZ" through (26.6476, 0, 380) normal (1, 0, 0) x (0, 0, -1)
ref_plane "to_Bolt_1_446_ZX" through (26.6476, 0, 380) normal (0, 0, -1) x (0, 1, 0)
ref_plane "to_Bolt_1_447_XY" through (28.3668, 0, 380) normal (0, 1, 0) x (1, 0, 0)
ref_plane "to_Bolt_1_447_YZ" through (28.3668, 0, 380) normal (1, 0, 0) x (0, 0, -1)
ref_plane "to_Bolt_1_447_ZX" through (28.3668, 0, 380) normal (0, 0, -1) x (0, 1, 0)
ref_plane "to_Bolt_1_448_XY" through (30.086, 0, 380) normal (0, 1, 0) x (1, 0, 0)
ref_plane "to_Bolt_1_448_YZ" through (30.086, 0, 380) normal (1, 0, 0) x (0, 0, -1)
ref_plane "to_Bolt_1_448_ZX" through (30.086, 0, 380) normal (0, 0, -1) x (0, 1, 0)
ref_plane "to_Bolt_1_449_XY" through (31.8052, 0, 380) normal (0, 1, 0) x (1, 0, 0)
ref_plane "to_Bolt_1_449_YZ" through (31.8052, 0, 380) normal (1, 0, 0) x (0, 0, -1)
ref_plane "to_Bolt_1_449_ZX" through (31.8052, 0, 380) normal (0, 0, -1) x (0, 1, 0)
ref_plane "to_Bolt_1_45_XY" through (-224.3553, 0, -380) normal (0, 1, 0) x (1, 0, 0)
ref_plane "to_Bolt_1_45_YZ" through (-224.3553, 0, -380) normal (1, 0, 0) x (0, 0, -1)
ref_plane "to_Bolt_1_45_ZX" through (-224.3553, 0, -380) normal (0, 0, -1) x (0, 1, 0)
ref_plane "to_Bolt_1_450_XY" through (33.5244, 0, 380) normal (0, 1, 0) x (1, 0, 0)
ref_plane "to_Bolt_1_450_YZ" through (33.5244, 0, 380) normal (1, 0, 0) x (0, 0, -1)
ref_plane "to_Bolt_1_450_ZX" through (33.5244, 0, 380) normal (0, 0, -1) x (0, 1, 0)
ref_plane "to_Bolt_1_451_XY" through (35.2436, 0, 380) normal (0, 1, 0) x (1, 0, 0)
ref_plane "to_Bolt_1_451_YZ" through (35.2436, 0, 380) normal (1, 0, 0) x (0, 0, -1)
ref_plane "to_Bolt_1_451_ZX" through (35.2436, 0, 380) normal (0, 0, -1) x (0, 1, 0)
ref_plane "to_Bolt_1_452_XY" through (36.9628, 0, 380) normal (0, 1, 0) x (1, 0, 0)
ref_plane "to_Bolt_1_452_YZ" through (36.9628, 0, 380) normal (1, 0, 0) x (0, 0, -1)
ref_plane "to_Bolt_1_452_ZX" through (36.9628, 0, 380) normal (0, 0, -1) x (0, 1, 0)
ref_plane "to_Bolt_1_453_XY" through (38.6819, 0, 380) normal (0, 1, 0) x (1, 0, 0)
ref_plane "to_Bolt_1_453_YZ" through (38.6819, 0, 380) normal (1, 0, 0) x (0, 0, -1)
ref_plane "to_Bolt_1_453_ZX" through (38.6819, 0, 380) normal (0, 0, -1) x (0, 1, 0)
ref_plane "to_Bolt_1_454_XY" through (40.4011, 0, 380) normal (0, 1, 0) x (1, 0, 0)
ref_plane "to_Bolt_1_454_YZ" through (40.4011, 0, 380) normal (1, 0, 0) x (0, 0, -1)
ref_plane "to_Bolt_1_454_ZX" through (40.4011, 0, 380) normal (0, 0, -1) x (0, 1, 0)
ref_plane "to_Bolt_1_455_XY" through (42.1203, 0, 380) normal (0, 1, 0) x (1, 0, 0)
ref_plane "to_Bolt_1_455_YZ" through (42.1203, 0, 380) normal (1, 0, 0) x (0, 0, -1)
ref_plane "to_Bolt_1_455_ZX" through (42.1203, 0, 380) normal (0, 0, -1) x (0, 1, 0)
ref_plane "to_Bolt_1_456_XY" through (43.8395, 0, 380) normal (0, 1, 0) x (1, 0, 0)
ref_plane "to_Bolt_1_456_YZ" through (43.8395, 0, 380) normal (1, 0, 0) x (0, 0, -1)
ref_plane "to_Bolt_1_456_ZX" through (43.8395, 0, 380) normal (0, 0, -1) x (0, 1, 0)
ref_plane "to_Bolt_1_457_XY" through (45.5587, 0, 380) normal (0, 1, 0) x (1, 0, 0)
ref_plane "to_Bolt_1_457_YZ" through (45.5587, 0, 380) normal (1, 0, 0) x (0, 0, -1)
ref_plane "to_Bolt_1_457_ZX" through (45.5587, 0, 380) normal (0, 0, -1) x (0, 1, 0)
ref_plane "to_Bolt_1_458_XY" through (47.2779, 0, 380) normal (0, 1, 0) x (1, 0, 0)
ref_plane "to_Bolt_1_458_YZ" through (47.2779, 0, 380) normal (1, 0, 0) x (0, 0, -1)
ref_plane "to_Bolt_1_458_ZX" through (47.2779, 0, 380) normal (0, 0, -1) x (0, 1, 0)
ref_plane "to_Bolt_1_459_XY" through (48.9971, 0, 380) normal (0, 1, 0) x (1, 0, 0)
ref_plane "to_Bolt_1_459_YZ" through (48.9971, 0, 380) normal (1, 0, 0) x (0, 0, -1)
ref_plane "to_Bolt_1_459_ZX" through (48.9971, 0, 380) normal (0, 0, -1) x (0, 1, 0)
ref_plane "to_Bolt_1_46_XY" through (-222.6361, 0, -380) normal (0, 1, 0) x (1, 0, 0)
ref_plane "to_Bolt_1_46_YZ" through (-222.6361, 0, -380) normal (1, 0, 0) x (0, 0, -1)
ref_plane "to_Bolt_1_46_ZX" through (-222.6361, 0, -380) normal (0, 0, -1) x (0, 1, 0)
ref_plane "to_Bolt_1_460_XY" through (50.7163, 0, 380) normal (0, 1, 0) x (1, 0, 0)
ref_plane "to_Bolt_1_460_YZ" through (50.7163, 0, 380) normal (1, 0, 0) x (0, 0, -1)
ref_plane "to_Bolt_1_460_ZX" through (50.7163, 0, 380) normal (0, 0, -1) x (0, 1, 0)
ref_plane "to_Bolt_1_461_XY" through (52.4355, 0, 380) normal (0, 1, 0) x (1, 0, 0)
ref_plane "to_Bolt_1_461_YZ" through (52.4355, 0, 380) normal (1, 0, 0) x (0, 0, -1)
ref_plane "to_Bolt_1_461_ZX" through (52.4355, 0, 380) normal (0, 0, -1) x (0, 1, 0)
ref_plane "to_Bolt_1_462_XY" through (54.1547, 0, 380) normal (0, 1, 0) x (1, 0, 0)
ref_plane "to_Bolt_1_462_YZ" through (54.1547, 0, 380) normal (1, 0, 0) x (0, 0, -1)
ref_plane "to_Bolt_1_462_ZX" through (54.1547, 0, 380) normal (0, 0, -1) x (0, 1, 0)
ref_plane "to_Bolt_1_463_XY" through (55.8739, 0, 380) normal (0, 1, 0) x (1, 0, 0)
ref_plane "to_Bolt_1_463_YZ" through (55.8739, 0, 380) normal (1, 0, 0) x (0, 0, -1)
ref_plane "to_Bolt_1_463_ZX" through (55.8739, 0, 380) normal (0, 0, -1) x (0, 1, 0)
ref_plane "to_Bolt_1_464_XY" through (57.5931, 0, 380) normal (0, 1, 0) x (1, 0, 0)
ref_plane "to_Bolt_1_464_YZ" through (57.5931, 0, 380) normal (1, 0, 0) x (0, 0, -1)
ref_plane "to_Bolt_1_464_ZX" through (57.5931, 0, 380) normal (0, 0, -1) x (0, 1, 0)
ref_plane "to_Bolt_1_465_XY" through (59.3123, 0, 380) normal (0, 1, 0) x (1, 0, 0)
ref_plane "to_Bolt_1_465_YZ" through (59.3123, 0, 380) normal (1, 0, 0) x (0, 0, -1)
ref_plane "to_Bolt_1_465_ZX" through (59.3123, 0, 380) normal (0, 0, -1) x (0, 1, 0)
ref_plane "to_Bolt_1_466_XY" through (61.0315, 0, 380) normal (0, 1, 0) x (1, 0, 0)
ref_plane "to_Bolt_1_466_YZ" through (61.0315, 0, 380) normal (1, 0, 0) x (0, 0, -1)
ref_plane "to_Bolt_1_466_ZX" through (61.0315, 0, 380) normal (0, 0, -1) x (0, 1, 0)
ref_plane "to_Bolt_1_467_XY" through (62.7507, 0, 380) normal (0, 1, 0) x (1, 0, 0)
ref_plane "to_Bolt_1_467_YZ" through (62.7507, 0, 380) normal (1, 0, 0) x (0, 0, -1)
ref_plane "to_Bolt_1_467_ZX" through (62.7507, 0, 380) normal (0, 0, -1) x (0, 1, 0)
ref_plane "to_Bolt_1_468_XY" through (64.4699, 0, 380) normal (0, 1, 0) x (1, 0, 0)
ref_plane "to_Bolt_1_468_YZ" through (64.4699, 0, 380) normal (1, 0, 0) x (0, 0, -1)
ref_plane "to_Bolt_1_468_ZX" through (64.4699, 0, 380) normal (0, 0, -1) x (0, 1, 0)
ref_plane "to_Bolt_1_469_XY" through (66.1891, 0, 380) normal (0, 1, 0) x (1, 0, 0)
ref_plane "to_Bolt_1_469_YZ" through (66.1891, 0, 380) normal (1, 0, 0) x (0, 0, -1)
ref_plane "to_Bolt_1_469_ZX" through (66.1891, 0, 380) normal (0, 0, -1) x (0, 1, 0)
ref_plane "to_Bolt_1_47_XY" through (-220.9169, 0, -380) normal (0, 1, 0) x (1, 0, 0)
ref_plane "to_Bolt_1_47_YZ" through (-220.9169, 0, -380) normal (1, 0, 0) x (0, 0, -1)
ref_plane "to_Bolt_1_47_ZX" through (-220.9169, 0, -380) normal (0, 0, -1) x (0, 1, 0)
ref_plane "to_Bolt_1_470_XY" through (67.9083, 0, 380) normal (0, 1, 0) x (1, 0, 0)
ref_plane "to_Bolt_1_470_YZ" through (67.9083, 0, 380) normal (1, 0, 0) x (0, 0, -1)
ref_plane "to_Bolt_1_470_ZX" through (67.9083, 0, 380) normal (0, 0, -1) x (0, 1, 0)
ref_plane "to_Bolt_1_471_XY" through (69.6275, 0, 380) normal (0, 1, 0) x (1, 0, 0)
ref_plane "to_Bolt_1_471_YZ" through (69.6275, 0, 380) normal (1, 0, 0) x (0, 0, -1)
ref_plane "to_Bolt_1_471_ZX" through (69.6275, 0, 380) normal (0, 0, -1) x (0, 1, 0)
ref_plane "to_Bolt_1_472_XY" through (71.3467, 0, 380) normal (0, 1, 0) x (1, 0, 0)
ref_plane "to_Bolt_1_472_YZ" through (71.3467, 0, 380) normal (1, 0, 0) x (0, 0, -1)
ref_plane "to_Bolt_1_472_ZX" through (71.3467, 0, 380) normal (0, 0, -1) x (0, 1, 0)
ref_plane "to_Bolt_1_473_XY" through (73.0659, 0, 380) normal (0, 1, 0) x (1, 0, 0)
ref_plane "to_Bolt_1_473_YZ" through (73.0659, 0, 380) normal (1, 0, 0) x (0, 0, -1)
ref_plane "to_Bolt_1_473_ZX" through (73.0659, 0, 380) normal (0, 0, -1) x (0, 1, 0)
ref_plane "to_Bolt_1_474_XY" through (74.7851, 0, 380) normal (0, 1, 0) x (1, 0, 0)
ref_plane "to_Bolt_1_474_YZ" through (74.7851, 0, 380) normal (1, 0, 0) x (0, 0, -1)
ref_plane "to_Bolt_1_474_ZX" through (74.7851, 0, 380) normal (0, 0, -1) x (0, 1, 0)
ref_plane "to_Bolt_1_475_XY" through (76.5043, 0, 380) normal (0, 1, 0) x (1, 0, 0)
ref_plane "to_Bolt_1_475_YZ" through (76.5043, 0, 380) normal (1, 0, 0) x (0, 0, -1)
ref_plane "to_Bolt_1_475_ZX" through (76.5043, 0, 380) normal (0, 0, -1) x (0, 1, 0)
ref_plane "to_Bolt_1_476_XY" through (78.2235, 0, 380) normal (0, 1, 0) x (1, 0, 0)
ref_plane "to_Bolt_1_476_YZ" through (78.2235, 0, 380) normal (1, 0, 0) x (0, 0, -1)
ref_plane "to_Bolt_1_476_ZX" through (78.2235, 0, 380) normal (0, 0, -1) x (0, 1, 0)
ref_plane "to_Bolt_1_477_XY" through (79.9427, 0, 380) normal (0, 1, 0) x (1, 0, 0)
ref_plane "to_Bolt_1_477_YZ" through (79.9427, 0, 380) normal (1, 0, 0) x (0, 0, -1)
ref_plane "to_Bolt_1_477_ZX" through (79.9427, 0, 380) normal (0, 0, -1) x (0, 1, 0)
ref_plane "to_Bolt_1_478_XY" through (81.6619, 0, 380) normal (0, 1, 0) x (1, 0, 0)
ref_plane "to_Bolt_1_478_YZ" through (81.6619, 0, 380) normal (1, 0, 0) x (0, 0, -1)
ref_plane "to_Bolt_1_478_ZX" through (81.6619, 0, 380) normal (0, 0, -1) x (0, 1, 0)
ref_plane "to_Bolt_1_479_XY" through (83.3811, 0, 380) normal (0, 1, 0) x (1, 0, 0)
ref_plane "to_Bolt_1_479_YZ" through (83.3811, 0, 380) normal (1, 0, 0) x (0, 0, -1)
ref_plane "to_Bolt_1_479_ZX" through (83.3811, 0, 380) normal (0, 0, -1) x (0, 1, 0)
ref_plane "to_Bolt_1_48_XY" through (-219.1977, 0, -380) normal (0, 1, 0) x (1, 0, 0)
ref_plane "to_Bolt_1_48_YZ" through (-219.1977, 0, -380) normal (1, 0, 0) x (0, 0, -1)
ref_plane "to_Bolt_1_48_ZX" through (-219.1977, 0, -380) normal (0, 0, -1) x (0, 1, 0)
ref_plane "to_Bolt_1_480_XY" through (85.1003, 0, 380) normal (0, 1, 0) x (1, 0, 0)
ref_plane "to_Bolt_1_480_YZ" through (85.1003, 0, 380) normal (1, 0, 0) x (0, 0, -1)
ref_plane "to_Bolt_1_480_ZX" through (85.1003, 0, 380) normal (0, 0, -1) x (0, 1, 0)
ref_plane "to_Bolt_1_481_XY" through (86.8195, 0, 380) normal (0, 1, 0) x (1, 0, 0)
ref_plane "to_Bolt_1_481_YZ" through (86.8195, 0, 380) normal (1, 0, 0) x (0, 0, -1)
ref_plane "to_Bolt_1_481_ZX" through (86.8195, 0, 380) normal (0, 0, -1) x (0, 1, 0)
ref_plane "to_Bolt_1_482_XY" through (88.5387, 0, 380) normal (0, 1, 0) x (1, 0, 0)
ref_plane "to_Bolt_1_482_YZ" through (88.5387, 0, 380) normal (1, 0, 0) x (0, 0, -1)
ref_plane "to_Bolt_1_482_ZX" through (88.5387, 0, 380) normal (0, 0, -1) x (0, 1, 0)
ref_plane "to_Bolt_1_483_XY" through (90.2579, 0, 380) normal (0, 1, 0) x (1, 0, 0)
ref_plane "to_Bolt_1_483_YZ" through (90.2579, 0, 380) normal (1, 0, 0) x (0, 0, -1)
ref_plane "to_Bolt_1_483_ZX" through (90.2579, 0, 380) normal (0, 0, -1) x (0, 1, 0)
ref_plane "to_Bolt_1_484_XY" through (91.9771, 0, 380) normal (0, 1, 0) x (1, 0, 0)
ref_plane "to_Bolt_1_484_YZ" through (91.9771, 0, 380) normal (1, 0, 0) x (0, 0, -1)
ref_plane "to_Bolt_1_484_ZX" through (91.9771, 0, 380) normal (0, 0, -1) x (0, 1, 0)
ref_plane "to_Bolt_1_485_XY" through (93.6963, 0, 380) normal (0, 1, 0) x (1, 0, 0)
ref_plane "to_Bolt_1_485_YZ" through (93.6963, 0, 380) normal (1, 0, 0) x (0, 0, -1)
ref_plane "to_Bolt_1_485_ZX" through (93.6963, 0, 380) normal (0, 0, -1) x (0, 1, 0)
ref_plane "to_Bolt_1_486_XY" through (95.4155, 0, 380) normal (0, 1, 0) x (1, 0, 0)
ref_plane "to_Bolt_1_486_YZ" through (95.4155, 0, 380) normal (1, 0, 0) x (0, 0, -1)
ref_plane "to_Bolt_1_486_ZX" through (95.4155, 0, 380) normal (0, 0, -1) x (0, 1, 0)
ref_plane "to_Bolt_1_487_XY" through (97.1347, 0, 380) normal (0, 1, 0) x (1, 0, 0)
ref_plane "to_Bolt_1_487_YZ" through (97.1347, 0, 380) normal (1, 0, 0) x (0, 0, -1)
ref_plane "to_Bolt_1_487_ZX" through (97.1347, 0, 380) normal (0, 0, -1) x (0, 1, 0)
ref_plane "to_Bolt_1_488_XY" through (98.8539, 0, 380) normal (0, 1, 0) x (1, 0, 0)
ref_plane "to_Bolt_1_488_YZ" through (98.8539, 0, 380) normal (1, 0, 0) x (0, 0, -1)
ref_plane "to_Bolt_1_488_ZX" through (98.8539, 0, 380) normal (0, 0, -1) x (0, 1, 0)
ref_plane "to_Bolt_1_489_XY" through (100.5731, 0, 380) normal (0, 1, 0) x (1, 0, 0)
ref_plane "to_Bolt_1_489_YZ" through (100.5731, 0, 380) normal (1, 0, 0) x (0, 0, -1)
ref_plane "to_Bolt_1_489_ZX" through (100.5731, 0, 380) normal (0, 0, -1) x (0, 1, 0)
ref_plane "to_Bolt_1_49_XY" through (-217.4785, 0, -380) normal (0, 1, 0) x (1, 0, 0)
ref_plane "to_Bolt_1_49_YZ" through (-217.4785, 0, -380) normal (1, 0, 0) x (0, 0, -1)
ref_plane "to_Bolt_1_49_ZX" through (-217.4785, 0, -380) normal (0, 0, -1) x (0, 1, 0)
ref_plane "to_Bolt_1_490_XY" through (102.2923, 0, 380) normal (0, 1, 0) x (1, 0, 0)
ref_plane "to_Bolt_1_490_YZ" through (102.2923, 0, 380) normal (1, 0, 0) x (0, 0, -1)
ref_plane "to_Bolt_1_490_ZX" through (102.2923, 0, 380) normal (0, 0, -1) x (0, 1, 0)
ref_plane "to_Bolt_1_491_XY" through (104.0115, 0, 380) normal (0, 1, 0) x (1, 0, 0)
ref_plane "to_Bolt_1_491_YZ" through (104.0115, 0, 380) normal (1, 0, 0) x (0, 0, -1)
ref_plane "to_Bolt_1_491_ZX" through (104.0115, 0, 380) normal (0, 0, -1) x (0, 1, 0)
ref_plane "to_Bolt_1_492_XY" through (105.7307, 0, 380) normal (0, 1, 0) x (1, 0, 0)
ref_plane "to_Bolt_1_492_YZ" through (105.7307, 0, 380) normal (1, 0, 0) x (0, 0, -1)
ref_plane "to_Bolt_1_492_ZX" through (105.7307, 0, 380) normal (0, 0, -1) x (0, 1, 0)
ref_plane "to_Bolt_1_493_XY" through (107.4499, 0, 380) normal (0, 1, 0) x (1, 0, 0)
ref_plane "to_Bolt_1_493_YZ" through (107.4499, 0, 380) normal (1, 0, 0) x (0, 0, -1)
ref_plane "to_Bolt_1_493_ZX" through (107.4499, 0, 380) normal (0, 0, -1) x (0, 1, 0)
ref_plane "to_Bolt_1_494_XY" through (109.1691, 0, 380) normal (0, 1, 0) x (1, 0, 0)
ref_plane "to_Bolt_1_494_YZ" through (109.1691, 0, 380) normal (1, 0, 0) x (0, 0, -1)
ref_plane "to_Bolt_1_494_ZX" through (109.1691, 0, 380) normal (0, 0, -1) x (0, 1, 0)
ref_plane "to_Bolt_1_495_XY" through (110.8883, 0, 380) normal (0, 1, 0) x (1, 0, 0)
ref_plane "to_Bolt_1_495_YZ" through (110.8883, 0, 380) normal (1, 0, 0) x (0, 0, -1)
ref_plane "to_Bolt_1_495_ZX" through (110.8883, 0, 380) normal (0, 0, -1) x (0, 1, 0)
ref_plane "to_Bolt_1_496_XY" through (112.6074, 0, 380) normal (0, 1, 0) x (1, 0, 0)
ref_plane "to_Bolt_1_496_YZ" through (112.6074, 0, 380) normal (1, 0, 0) x (0, 0, -1)
ref_plane "to_Bolt_1_496_ZX" through (112.6074, 0, 380) normal (0, 0, -1) x (0, 1, 0)
ref_plane "to_Bolt_1_497_XY" through (114.3266, 0, 380) normal (0, 1, 0) x (1, 0, 0)
ref_plane "to_Bolt_1_497_YZ" through (114.3266, 0, 380) normal (1, 0, 0) x (0, 0, -1)
ref_plane "to_Bolt_1_497_ZX" through (114.3266, 0, 380) normal (0, 0, -1) x (0, 1, 0)
ref_plane "to_Bolt_1_498_XY" through (116.0458, 0, 380) normal (0, 1, 0) x (1, 0, 0)
ref_plane "to_Bolt_1_498_YZ" through (116.0458, 0, 380) normal (1, 0, 0) x (0, 0, -1)
ref_plane "to_Bolt_1_498_ZX" through (116.0458, 0, 380) normal (0, 0, -1) x (0, 1, 0)
ref_plane "to_Bolt_1_499_XY" through (117.765, 0, 380) normal (0, 1, 0) x (1, 0, 0)
ref_plane "to_Bolt_1_499_YZ" through (117.765, 0, 380) normal (1, 0, 0) x (0, 0, -1)
ref_plane "to_Bolt_1_499_ZX" through (117.765, 0, 380) normal (0, 0, -1) x (0, 1, 0)
ref_plane "to_Bolt_1_5_XY" through (-293.1232, 0, -380) normal (0, 1, 0) x (1, 0, 0)
ref_plane "to_Bolt_1_5_YZ" through (-293.1232, 0, -380) normal (1, 0, 0) x (0, 0, -1)
ref_plane "to_Bolt_1_5_ZX" through (-293.1232, 0, -380) normal (0, 0, -1) x (0, 1, 0)
ref_plane "to_Bolt_1_50_XY" through (-215.7593, 0, -380) normal (0, 1, 0) x (1, 0, 0)
ref_plane "to_Bolt_1_50_YZ" through (-215.7593, 0, -380) normal (1, 0, 0) x (0, 0, -1)
ref_plane "to_Bolt_1_50_ZX" through (-215.7593, 0, -380) normal (0, 0, -1) x (0, 1, 0)
ref_plane "to_Bolt_1_500_XY" through (119.4842, 0, 380) normal (0, 1, 0) x (1, 0, 0)
ref_plane "to_Bolt_1_500_YZ" through (119.4842, 0, 380) normal (1, 0, 0) x (0, 0, -1)
ref_plane "to_Bolt_1_500_ZX" through (119.4842, 0, 380) normal (0, 0, -1) x (0, 1, 0)
ref_plane "to_Bolt_1_501_XY" through (121.2034, 0, 380) normal (0, 1, 0) x (1, 0, 0)
ref_plane "to_Bolt_1_501_YZ" through (121.2034, 0, 380) normal (1, 0, 0) x (0, 0, -1)
ref_plane "to_Bolt_1_501_ZX" through (121.2034, 0, 380) normal (0, 0, -1) x (0, 1, 0)
ref_plane "to_Bolt_1_502_XY" through (122.9226, 0, 380) normal (0, 1, 0) x (1, 0, 0)
ref_plane "to_Bolt_1_502_YZ" through (122.9226, 0, 380) normal (1, 0, 0) x (0, 0, -1)
ref_plane "to_Bolt_1_502_ZX" through (122.9226, 0, 380) normal (0, 0, -1) x (0, 1, 0)
ref_plane "to_Bolt_1_503_XY" through (124.6418, 0, 380) normal (0, 1, 0) x (1, 0, 0)
ref_plane "to_Bolt_1_503_YZ" through (124.6418, 0, 380) normal (1, 0, 0) x (0, 0, -1)
ref_plane "to_Bolt_1_503_ZX" through (124.6418, 0, 380) normal (0, 0, -1) x (0, 1, 0)
ref_plane "to_Bolt_1_504_XY" through (126.361, 0, 380) normal (0, 1, 0) x (1, 0, 0)
ref_plane "to_Bolt_1_504_YZ" through (126.361, 0, 380) normal (1, 0, 0) x (0, 0, -1)
ref_plane "to_Bolt_1_504_ZX" through (126.361, 0, 380) normal (0, 0, -1) x (0, 1, 0)
ref_plane "to_Bolt_1_505_XY" through (128.0802, 0, 380) normal (0, 1, 0) x (1, 0, 0)
ref_plane "to_Bolt_1_505_YZ" through (128.0802, 0, 380) normal (1, 0, 0) x (0, 0, -1)
ref_plane "to_Bolt_1_505_ZX" through (128.0802, 0, 380) normal (0, 0, -1) x (0, 1, 0)
ref_plane "to_Bolt_1_506_XY" through (129.7994, 0, 380) normal (0, 1, 0) x (1, 0, 0)
ref_plane "to_Bolt_1_506_YZ" through (129.7994, 0, 380) normal (1, 0, 0) x (0, 0, -1)
ref_plane "to_Bolt_1_506_ZX" through (129.7994, 0, 380) normal (0, 0, -1) x (0, 1, 0)
ref_plane "to_Bolt_1_507_XY" through (131.5186, 0, 380) normal (0, 1, 0) x (1, 0, 0)
ref_plane "to_Bolt_1_507_YZ" through (131.5186, 0, 380) normal (1, 0, 0) x (0, 0, -1)
ref_plane "to_Bolt_1_507_ZX" through (131.5186, 0, 380) normal (0, 0, -1) x (0, 1, 0)
ref_plane "to_Bolt_1_508_XY" through (133.2378, 0, 380) normal (0, 1, 0) x (1, 0, 0)
ref_plane "to_Bolt_1_508_YZ" through (133.2378, 0, 380) normal (1, 0, 0) x (0, 0, -1)
ref_plane "to_Bolt_1_508_ZX" through (133.2378, 0, 380) normal (0, 0, -1) x (0, 1, 0)
ref_plane "to_Bolt_1_509_XY" through (134.957, 0, 380) normal (0, 1, 0) x (1, 0, 0)
ref_plane "to_Bolt_1_509_YZ" through (134.957, 0, 380) normal (1, 0, 0) x (0, 0, -1)
ref_plane "to_Bolt_1_509_ZX" through (134.957, 0, 380) normal (0, 0, -1) x (0, 1, 0)
ref_plane "to_Bolt_1_51_XY" through (-214.0401, 0, -380) normal (0, 1, 0) x (1, 0, 0)
ref_plane "to_Bolt_1_51_YZ" through (-214.0401, 0, -380) normal (1, 0, 0) x (0, 0, -1)
ref_plane "to_Bolt_1_51_ZX" through (-214.0401, 0, -380) normal (0, 0, -1) x (0, 1, 0)
ref_plane "to_Bolt_1_510_XY" through (136.6762, 0, 380) normal (0, 1, 0) x (1, 0, 0)
ref_plane "to_Bolt_1_510_YZ" through (136.6762, 0, 380) normal (1, 0, 0) x (0, 0, -1)
ref_plane "to_Bolt_1_510_ZX" through (136.6762, 0, 380) normal (0, 0, -1) x (0, 1, 0)
ref_plane "to_Bolt_1_52_XY" through (-212.3209, 0, -380) normal (0, 1, 0) x (1, 0, 0)
ref_plane "to_Bolt_1_52_YZ" through (-212.3209, 0, -380) normal (1, 0, 0) x (0, 0, -1)
ref_plane "to_Bolt_1_52_ZX" through (-212.3209, 0, -380) normal (0, 0, -1) x (0, 1, 0)
ref_plane "to_Bolt_1_53_XY" through (-210.6017, 0, -380) normal (0, 1, 0) x (1, 0, 0)
ref_plane "to_Bolt_1_53_YZ" through (-210.6017, 0, -380) normal (1, 0, 0) x (0, 0, -1)
ref_plane "to_Bolt_1_53_ZX" through (-210.6017, 0, -380) normal (0, 0, -1) x (0, 1, 0)
ref_plane "to_Bolt_1_54_XY" through (-208.8825, 0, -380) normal (0, 1, 0) x (1, 0, 0)
ref_plane "to_Bolt_1_54_YZ" through (-208.8825, 0, -380) normal (1, 0, 0) x (0, 0, -1)
ref_plane "to_Bolt_1_54_ZX" through (-208.8825, 0, -380) normal (0, 0, -1) x (0, 1, 0)
ref_plane "to_Bolt_1_55_XY" through (-207.1633, 0, -380) normal (0, 1, 0) x (1, 0, 0)
ref_plane "to_Bolt_1_55_YZ" through (-207.1633, 0, -380) normal (1, 0, 0) x (0, 0, -1)
ref_plane "to_Bolt_1_55_ZX" through (-207.1633, 0, -380) normal (0, 0, -1) x (0, 1, 0)
ref_plane "to_Bolt_1_56_XY" through (-205.4441, 0, -380) normal (0, 1, 0) x (1, 0, 0)
ref_plane "to_Bolt_1_56_YZ" through (-205.4441, 0, -380) normal (1, 0, 0) x (0, 0, -1)
ref_plane "to_Bolt_1_56_ZX" through (-205.4441, 0, -380) normal (0, 0, -1) x (0, 1, 0)
ref_plane "to_Bolt_1_57_XY" through (-203.7249, 0, -380) normal (0, 1, 0) x (1, 0, 0)
ref_plane "to_Bolt_1_57_YZ" through (-203.7249, 0, -380) normal (1, 0, 0) x (0, 0, -1)
ref_plane "to_Bolt_1_57_ZX" through (-203.7249, 0, -380) normal (0, 0, -1) x (0, 1, 0)
ref_plane "to_Bolt_1_58_XY" through (-202.0057, 0, -380) normal (0, 1, 0) x (1, 0, 0)
ref_plane "to_Bolt_1_58_YZ" through (-202.0057, 0, -380) normal (1, 0, 0) x (0, 0, -1)
ref_plane "to_Bolt_1_58_ZX" through (-202.0057, 0, -380) normal (0, 0, -1) x (0, 1, 0)
ref_plane "to_Bolt_1_59_XY" through (-200.2865, 0, -380) normal (0, 1, 0) x (1, 0, 0)
ref_plane "to_Bolt_1_59_YZ" through (-200.2865, 0, -380) normal (1, 0, 0) x (0, 0, -1)
ref_plane "to_Bolt_1_59_ZX" through (-200.2865, 0, -380) normal (0, 0, -1) x (0, 1, 0)
ref_plane "to_Bolt_1_6_XY" through (-291.404, 0, -380) normal (0, 1, 0) x (1, 0, 0)